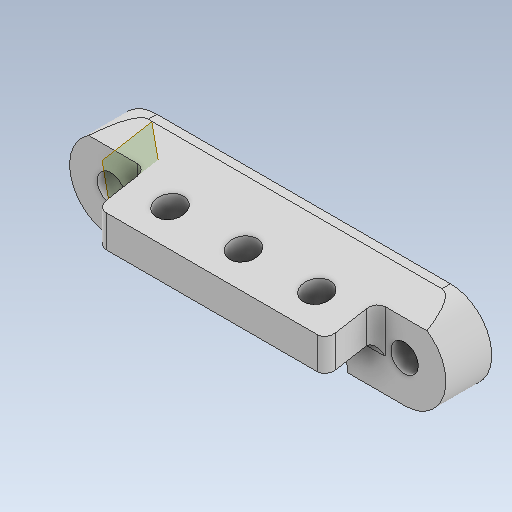
# Autodesk Inventor part: pcb_shell_n1
Saved by Autodesk Inventor 2020 (Build 240168000, 168)
## iProperties
Created: 2019-08-29
Part Number: pcb_shell_n1
Material: Generic
Document SubType Name: Modeling
Designer: psrob
Density: 1 g/cm^3
Appearance: Default
Author: psrob
Autodesk Inventor part; units mm, degrees
ref_plane "YZ Plane" through (0, 0, 0) normal (1, 0, 0) x (0, 1, 0)
ref_plane "XZ Plane" through (0, 0, 0) normal (0, 1, 0) x (-1, 0, 0)
ref_plane "XY Plane" through (0, 0, 0) normal (0, 0, 1) x (1, 0, 0)
sketch "Sketch1" plane through (0, 0, 0) normal (0, 0, 1) x (1, 0, 0)
  circle A0 centre (4.5, 25.5) radius 1.5 projected
  circle A1 centre (-19.5, 25.5) radius 1.5 projected
  circle A2 centre (12.5, 25.5) radius 1.5 projected
  circle A3 centre (4.5, 33.5) radius 1.5 projected
  circle A4 centre (-19.5, 33.5) radius 1.5 projected
  circle A5 centre (12.5, 33.5) radius 1.5 projected
  arc A6 (-22, 39) -> (-24, 37) centre (-22, 37) ccw projected
  line L0 (-24, 1) -> (-24, 37) projected
  line L1 (-11, 1) -> (-24, 1) projected
  line L2 (-11, -3) -> (-11, 1) projected
  line L3 (-3, -3) -> (-11, -3) projected
  line L4 (-3, 1) -> (-3, -3) projected
  line L5 (18, 1) -> (-3, 1) projected
  line L6 (18, 1) -> (18, 37) projected
  arc A7 (18, 37) -> (16, 39) centre (16, 37) ccw projected
  line L7 (16, 39) -> (2, 39) projected
  arc A8 (2, 39) -> (0, 37) centre (2, 37) ccw projected
  line L8 (0, 7) -> (0, 37) projected
  arc A9 (-3, 4) -> (0, 7) centre (-3, 7) ccw projected
  line L9 (-11, 4) -> (-3, 4) projected
  arc A10 (-14, 7) -> (-11, 4) centre (-11, 7) ccw projected
  line L10 (-14, 7) -> (-14, 37) projected
  arc A11 (-14, 37) -> (-16, 39) centre (-16, 37) ccw projected
  line L11 (-16, 39) -> (-22, 39) projected
  circle A12 centre (-19.5, 14.5) radius 1.5 projected
  circle A13 centre (-19.5, 6.5) radius 1.5 projected
  circle A14 centre (12.5, 14.5) radius 1.5 projected
  circle A15 centre (12.5, 6.5) radius 1.5 projected
  circle A16 centre (4.5, 14.5) radius 1.5 projected
  circle A17 centre (4.5, 6.5) radius 1.5 projected
  circle A18 centre (-19.5, 6.5) radius 4.5
  circle A19 centre (12.5, 6.5) radius 4.5
  line L12 (-19.5, 6.5) -> (-19.5, 11)
  line L13 (12.5, 6.5) -> (12.5, 11)
  line L14 (-19.5, 11) -> (12.5, 11)
  line L15 (12.5, 6.5) -> (12.5, 2)
  line L16 (-19.5, 6.5) -> (-19.5, 2)
  line L17 (-19.5, 2) -> (12.5, 2)
  point P0 (0, 0)
  dimension "d0" = 9
  dimension "d1" = 9
  constraints: 12 end point, 4 point on circle, 2 centre point, 2 coincident, 2 point on line, 1 parallel, 1 vertical
  measures "d0" diameter of A18
  measures "d1" diameter of A19
extrude "Extrusion1" add sketch "Sketch1" along normal blind 5 contours A18 L12 A13 L16 | L14 L10 A10 L9 A9 L8 A19 L17 A18 | A18 L16 A13 L12 | L14 L8 A9 L9 A10 L10 | L15 A15 L13 A19 | A19 L13 A15 L15
sketch "Sketch2" plane through (0, 0, 5) normal (0, 0, 1) x (1, 0, 0)
  circle A0 centre (4.5, 6.5) radius 1.5 projected
  point P0 (0, 0)
extrude "Extrusion2" add sketch "Sketch2" against normal up to surface (5 mm away)
ref_plane "Work Plane1" through (-15.6225, 10.6368, 3) normal (-1, 0, 0) x (0, -0.1736482, 0.9848078)
sketch "Sketch3" plane through (-15.6225, 10.6368, 3) normal (-1, 0, 0) x (0, -0.1736482, 0.9848078)
  line L0 (1, 0) -> (1, 3) projected
  line L1 (6, 0) -> (1, 0) projected
  line L2 (6, 3) -> (6, 0) projected
  line L3 (1, 3) -> (6, 3) projected
  line L4 (6, 0) -> (7.5, 0)
  line L5 (3.4694, -8.1583) -> (1.9065, 0.705) projected
  line L6 (7.5, 0) -> (8.1078, -3.4468)
  line L7 (8.1078, -3.4468) -> (2.6386, -3.4468)
  point P0 (-1.1074, -10.9961)
  point P1 (2.0309, 0)
  dimension "d6" = 1.5
  dimension "d7" = 3.5
  constraints: 6 end point, 2 parallel, 1 horizontal, 1 point on line
  measures "d6" distance of L1.start L4.end
  measures "d7" distance of L4.end L6.end
ref_plane "Work Plane2" through (9.3775, 9.5949, 3.9848) normal (1, 0, 0) x (0, 0.9848078, 0.1736482)
extrude "Extrusion3" add sketch "Sketch3" against normal up to surface (25 mm away) contours L1 L4 L6 L7 L5
sketch "Sketch4" plane through (-15.6225, 10.6368, 3) normal (-1, 0, 0) x (0, -0.1736482, 0.9848078)
  line L0 (2.6386, -3.4468) -> (8.1078, -3.4468) projected
  line L1 (8.1078, -3.4468) -> (7.5, 0) projected
  line L2 (7.5, 0) -> (2.0309, 0) projected
  line L3 (2.6386, -3.4468) -> (2.0309, 0) projected
  line L4 (-3.0175, -0.1632) -> (1.9065, 0.705) projected
  line L5 (3.4694, -8.1583) -> (1.9065, 0.705) projected
  line L6 (7.5, 0) -> (2.0309, 0) projected
  line L7 (2.0309, 0) -> (-7.9691, 0)
  line L8 (-7.9691, 0) -> (7.5, 0)
  line L9 (7.5, 0) -> (7.5, 2.5396)
  line L10 (7.5, 2.5396) -> (-7.9691, 2.5396)
  line L11 (-7.9691, 2.5396) -> (-7.9691, 0)
  point P0 (-1.1074, -10.9961)
  point P1 (-2.0917, 0)
  dimension "d10" = 10
  constraints: 10 end point, 2 parallel, 1 collinear, 1 horizontal, 1 perpendicular
  measures "d10" distance of L2.end L7.end
extrude "Extrusion4" cut sketch "Sketch4" along normal mid plane 200 contours L7 L4 L5
sketch "Sketch5" plane through (-19.5, 11, 0.9401) normal (0, 0.9848078, 0.1736482) x (1, 0, 0)
  circle A0 centre (8.3775, -6.0917) radius 1.5 projected
  circle A1 centre (16.3775, -6.0917) radius 1.5 projected
  circle A2 centre (24.3775, -6.0917) radius 1.5 projected
  point P0 (19.5, -0.9843)
extrude "Extrusion5" cut sketch "Sketch5" against normal blind 10
fillet "Fillet1" radius 1 8 edges at (-15.6225, 8.5341, 5) (-15.6225, 7.5844, 10.3861) (9.3775, 7.5844, 10.3861) (9.3775, 8.5341, 5) (-13.6874, 6.7841, 5) (-7.1225, 6.7841, 5) (0.8775, 6.7841, 5) (7.4424, 6.7841, 5)
body "Solid1"
